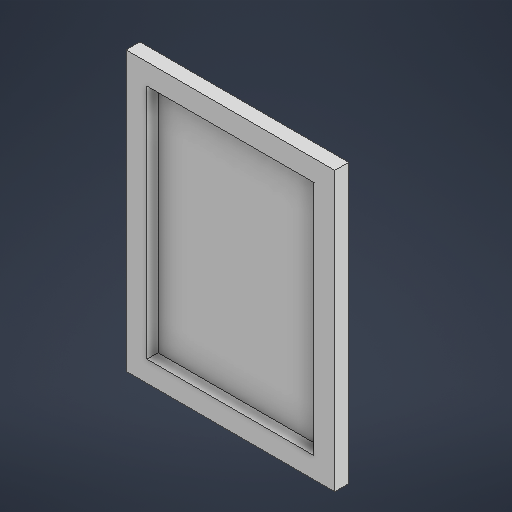
# Autodesk Inventor part: project1
Saved by Autodesk Inventor 2026 (Build 300175000, 175)
## iProperties
Created: 2026-09-08
Part Number: project1
Material: Типовые
Document SubType Name: Modeling
Designer: Roman
Density: 1 g/cm^3
Appearance: По умолчанию
Author: Roman
Autodesk Inventor part; units mm, degrees
ref_plane "YZ Plane" through (0, 0, 0) normal (1, 0, 0) x (0, 1, 0)
ref_plane "XZ Plane" through (0, 0, 0) normal (0, 1, 0) x (-1, 0, 0)
ref_plane "XY Plane" through (0, 0, 0) normal (0, 0, 1) x (1, 0, 0)
sketch "Эскиз3" plane through (0, 0, 0) normal (0, 0, 1) x (1, 0, 0)
  line L0 (75, -100) -> (-75, -100)
  line L1 (-75, -100) -> (-75, 100)
  line L2 (-75, 100) -> (75, 100)
  line L3 (75, 100) -> (75, -100)
  line L4 (75, -100) -> (-75, 100) construction
  line L5 (-75, -100) -> (75, 100) construction
  line L6 (-60, 85) -> (-60, -85)
  line L7 (-60, -85) -> (60, -85)
  line L8 (60, -85) -> (60, 85)
  line L9 (60, 85) -> (-60, 85)
  point P0 (0, 0)
  dimension "d11" = 150
  dimension "d12" = 200
  dimension "d13" = 15
  constraints: 20 end point, 4 parallel, 2 midpoint, 2 perpendicular, 1 horizontal, 3 other
  measures "d11" distance between parallel lines of L3 L1
  measures "d12" distance between parallel lines of L0 L2
  measures "d13" distance between parallel lines of L9 L2
extrude "Толщина рамки" add sketch "Эскиз3" along normal mid plane 10
sketch "Эскиз5" plane through (0, 0, 0) normal (1, 0, 0) x (0, 1, 0)
  line L0 (-100, -5) -> (100, -5) projected
  line L1 (0, -5) -> (-100, -31.7949)
  line L2 (-100, -31.7949) -> (-100, -5)
  line L3 (85, -5) -> (-85, -5) projected
  point P0 (0, 0)
  dimension "d16" = 15
  dimension "d24" = 100
  constraints: 4 end point, 1 midpoint, 1 perpendicular
  measures "d16" angle of L1 L0
  measures "d24" distance from line of L2 L1.start
extrude "Толищна подставки" add sketch "Эскиз5" along normal mid plane 20
sketch "Эскиз11" plane through (0, 0, -5) normal (0, 0, -1) x (-1, 0, 0)
  line L0 (-60, 85) -> (60, 85) projected
  line L1 (60, 85) -> (60, -85) projected
  line L2 (60, -85) -> (10, -85) projected
  line L3 (-10, -85) -> (-60, -85) projected
  line L4 (-60, -85) -> (-60, 85) projected
  line L5 (10, -85) -> (-10, -85) projected
  point P0 (0, 0)
extrude "Толщина зад. стенки" add sketch "Эскиз11" against normal blind 2
